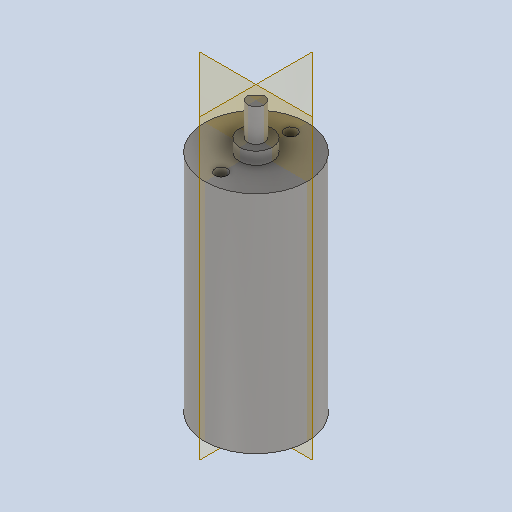
# Autodesk Inventor part: motor_small
Saved by Autodesk Inventor 2022.6 (Build 266554000, 554)
## iProperties
Created: 2024-10-11
Part Number: motor_small
Material: Iron, Malleable
Document SubType Name: Modeling
Designer: Zhong
Density: 7.15 g/cm^3
Appearance: Semi-Polished
Author: Zhong
Autodesk Inventor part; units mm, degrees
ref_plane "XZ Plane" through (0, 0, 0) normal (0, 1, 0) x (-1, 0, 0)
sketch "Sketch1" plane through (0, 0, 0) normal (0, 1, 0) x (-1, 0, 0)
  circle A0 centre (0, 0) radius 12.5
  dimension "d0" = 25
  constraints: 1 centre point, 1 coincident
  measures "d0" diameter of A0
extrude "Extrusion1" add sketch "Sketch1" along normal blind 55
sketch "Sketch2" plane through (0, 55, 0) normal (0, 1, 0) x (1, 0, 0)
  circle A0 centre (0, 0) radius 12.5 projected
  circle A1 centre (0, 0) radius 4
  dimension "d3" = 8
  constraints: 1 centre point, 1 coincident
  measures "d3" diameter of A1
extrude "Extrusion2" add sketch "Sketch2" along normal blind 3 contours A1
sketch "Sketch3" plane through (0, 58, 0) normal (0, 1, 0) x (1, 0, 0)
  circle A0 centre (0, 0) radius 4 projected
  circle A1 centre (0, 0) radius 2
  line L0 (-2, 0) -> (0.25, 1.9843)
  line L1 (-17.5, 0) -> (17.5, 0) projected
  dimension "d6" = 4
  dimension "d7" = 3
  constraints: 2 end point, 2 point on circle, 1 centre point, 1 coincident, 1 point on line
  measures "d6" diameter of A1
  measures "d7" distance of L0.start L0.end
extrude "Extrusion3" add sketch "Sketch3" along normal blind 8 contours L1 L0 A1 | A1 L1
sketch "Sketch4" plane through (0, 55, 0) normal (0, 1, 0) x (1, 0, 0)
  circle A0 centre (0, 0) radius 4 projected
  circle A1 centre (0, 0) radius 12.5 projected
  circle A2 centre (0, 0) radius 8.5 construction
  line L0 (-17.5, 0) -> (17.5, 0) construction
  line L1 (0, 17.5) -> (0, -17.5) construction
  point P0 (0, -8.5)
  point P1 (0, 8.5)
  dimension "d10" = 17
  constraints: 2 point on circle, 2 point on line, 1 centre point, 1 coincident
  measures "d10" diameter of A2
hole "Hole1" at (0, 55, -8.5) at (0, 55, 8.5) direction (0, -1, 0) diameter 3 depth 8 tip angle 118
body "Solid1"
